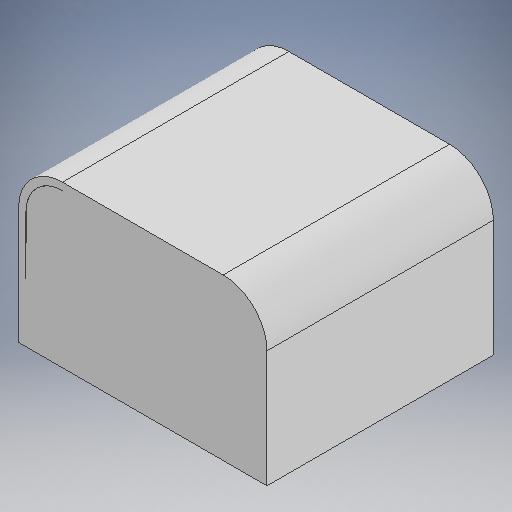
# Autodesk Inventor part: SERVO.housing
Saved by Autodesk Inventor 2025.3 (Build 293356000, 356)
## iProperties
Created: 2026-04-12
Part Number: SERVO.housing
Material: Generic
Document SubType Name: Modeling
Designer: user
Density: 1 g/cm^3
Appearance: Default
Author: user
## iProperties of the stored document SERVO.housing_3DPrint.ipt
Created: 2026-04-12
Part Number: SERVO.housing_3DPrint
Material: Generic
Document SubType Name: Modeling
Designer: user
Density: 1 g/cm^3
Appearance: Default
Author: user
Autodesk Inventor part; units mm, degrees
ref_plane "YZ Plane" through (0, 0, 0) normal (1, 0, 0) x (0, 1, 0)
ref_plane "XZ Plane" through (0, 0, 0) normal (0, 1, 0) x (-1, 0, 0)
sketch "Sketch1" plane through (0, 0, 0) normal (0, 0, 1) x (1, 0, 0)
  line L0 (11.1109, 10.667) -> (-10.8891, 10.667)
  arc A0 (17.1109, 4.667) -> (11.1109, 10.667) centre (11.1109, 4.667) ccw
  arc A1 (-10.8891, 10.667) -> (-16.8891, 4.667) centre (-10.8891, 4.667) ccw
  line L1 (17.1109, -11.333) -> (17.1109, 4.667)
  arc A2 (17.1109, 4.667) -> (11.1109, 10.667) centre (11.1109, 4.667) ccw
  line L2 (11.1109, 10.667) -> (-10.8891, 10.667)
  arc A3 (-10.8891, 10.667) -> (-16.8891, 4.667) centre (-10.8891, 4.667) ccw
  line L3 (-16.8891, 4.667) -> (-16.8891, -11.333)
  line L4 (16.1109, 4.667) -> (16.1109, -11.333)
  line L5 (17.1109, -11.333) -> (-16.8891, -11.333)
  line L6 (-15.8891, -11.333) -> (-15.8891, 4.667)
  arc A4 (-10.8891, 9.667) -> (-15.8891, 4.667) centre (-10.8891, 4.667) ccw
  line L7 (-10.8891, 9.667) -> (11.1109, 9.667)
  arc A5 (16.1109, 4.667) -> (11.1109, 9.667) centre (11.1109, 4.667) ccw
  line L8 (-16.8891, -3.333) -> (17.1109, -3.333)
  line L9 (-15.8891, -3.333) -> (-15.8891, 7.1792)
  line L10 (-15.8891, 2.667) -> (-13.8891, 2.667)
  line L11 (16.1109, -3.333) -> (-15.8891, -3.333)
  circle A6 centre (-13.8891, 2.667) radius 2
  line L12 (20.9541, 5.1792) -> (19.218, 5.1792)
  circle A7 centre (-13.8891, 2.667) radius 1.6
  line L13 (-13.8891, 4.267) -> (-15.8891, 4.267)
  line L14 (-15.8891, 4.267) -> (-15.8891, 1.067)
  line L15 (-15.8891, 1.067) -> (-13.8891, 1.067)
  line L16 (-13.8891, 1.067) -> (-13.8891, 4.267)
  circle A8 centre (13.4109, 2.667) radius 2
  circle A9 centre (13.4109, 2.667) radius 1.6
  line L17 (16.1109, 4.667) -> (16.1109, -3.333)
  line L18 (13.4109, 4.267) -> (16.1109, 4.267)
  line L19 (16.1109, 4.267) -> (16.1109, 1.267)
  line L20 (16.1109, 1.267) -> (13.4109, 1.267)
  line L21 (13.4109, 1.267) -> (13.4109, 4.267)
  point P0 (0, 0)
  point P1 (16.1109, -3.333)
  point P2 (-15.8891, -3.333)
  point P3 (17.1109, 4.667)
  point P4 (-16.8891, 4.667)
  point P5 (-13.8891, 2.667)
  point P6 (-15.8891, 1.067)
  point P7 (-15.0891, 1.067)
  point P8 (-15.0891, 4.267)
  point P9 (-15.8891, 4.267)
  point P10 (14.8392, 1.267)
  point P11 (16.1109, 1.267)
  point P12 (16.1109, 4.267)
  point P13 (14.6109, 4.267)
  dimension "d16" = 3.2
  dimension "d18" = 3.2
  dimension "d19" = 27.3
  dimension "d0" = 1
  dimension "d3" = 22
  dimension "d4" = 34
  dimension "d5" = 16
  dimension "d6" = 6
  dimension "d7" = 5
  dimension "d8" = 9.667
  dimension "d9" = 10.667
  dimension "d10" = 11.333
  dimension "d11" = 8
  dimension "d12" = 22
  dimension "d13" = 34
  dimension "d14" = 6
  dimension "d15" = 4
  dimension "d17" = 4
  dimension "d20" = 0
  dimension "d21" = 0
  constraints: 42 end point, 12 point on circle, 8 centre point, 7 parallel, 4 horizontal, 4 point on line, 3 coincident, 3 midpoint, 2 equal radius, 2 perpendicular, 2 vertical alignment, 1 horizontal alignment, 10 other
  measures "d0" distance between parallel lines of L1 L4
  measures "d3" distance of L0.start L0.end
  measures "d4" distance of L8.start L8.end
  measures "d5" distance of L5.start L1.end
  measures "d6" radius of A0
  measures "d7" radius of A5
  measures "d8" distance from line of point (0, 0) L7
  measures "d9" distance from line of point (0, 0) L0
  measures "d10" distance from line of point (0, 0) L5
  measures "d11" distance between parallel lines of L5 L8
  measures "d12" distance of A0.centre A1.centre
  measures "d13" distance between parallel lines of L3 L1
  measures "d14" distance between parallel lines of L11 L10
  measures "d15" diameter of A6
  measures "d17" diameter of A8
  measures "d20" distance between parallel lines of L6 L9
  measures "d21" distance between parallel lines of L8 L11
extrude "Extrusion1" add sketch "Sketch1" along normal blind 31 contours A0 L1 L8 L4 A5 L7 A4 L6 L3 A1 L0 | L1 L5 L4 L8 | L8 L6 L5 L3 | L4 L5 L6 L8
extrude "Extrusion2" add sketch "Sketch1" along normal blind 5 contours L20 A8 L18 L4 | L6 A6 L15 | L20 A9 L18 A8 | A8 L18 A9 L20 | A6 L13 A7 L10 | L6 L13 A6 | L10 A7 L15 A6 | L15 A7 L13 A6
ref_plane "Work Plane1" through (0, 0, 31) normal (0, 0, -1) x (-1, 0, 0)
sketch "Sketch2" plane through (0, 0, 31) normal (0, 0, 1) x (1, 0, 0)
  line L0 (-15.8891, -3.333) -> (-15.8891, 1.067) projected
  line L1 (-15.8891, -3.333) -> (-15.8891, 5)
  line L2 (16.1109, -3.333) -> (-15.8891, -3.333) projected
  line L3 (-15.8891, -3.333) -> (16.1109, -3.333)
  line L4 (16.1109, -3.333) -> (16.1109, 4.667)
  arc A0 (16.1109, 4.667) -> (11.1109, 9.667) centre (11.1109, 4.667) ccw projected
  circle A1 centre (11.1109, 4.667) radius 5
  circle A2 centre (-10.8708, 4.667) radius 5
  line L5 (-10.8708, 10.6741) -> (11.1109, 10.6741)
  line L6 (-10.8708, 9.667) -> (11.1109, 9.667)
  line L7 (-10.8708, 9.667) -> (11.1109, 9.667)
  line L8 (-15.8891, -3.333) -> (16.1109, -3.333)
  line L9 (16.1109, 4.667) -> (16.1109, -3.333)
  line L10 (-15.8891, -3.333) -> (-15.8708, 4.6784)
  point P0 (0, 0)
  dimension "d25" = 10
  constraints: 18 end point, 3 horizontal, 2 point on circle, 2 tangent, 1 centre point, 1 coincident, 1 collinear, 1 horizontal alignment, 1 perpendicular, 1 point on line, 1 vertical, 3 other
extrude "Extrusion3" add sketch "Sketch2" against normal blind 1
body "Solid1"
